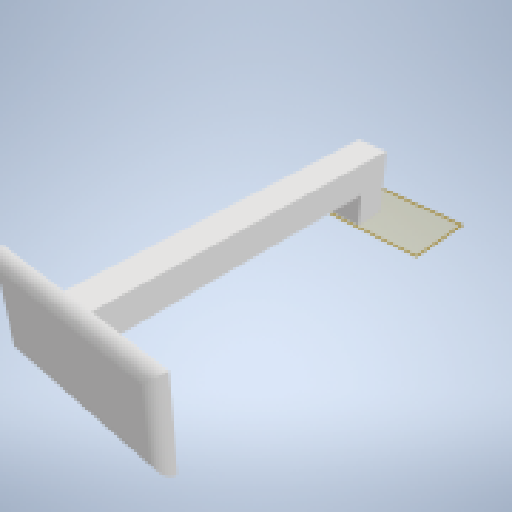
# Autodesk Inventor part: Part61
Saved by Autodesk Inventor 2023 (Build 270158000, 158)
## iProperties
Created: 2023-02-13
Part Number: Part61
Material: Generic
Document SubType Name: Modeling
Designer: klebe
Density: 1 g/cm^3
Appearance: Default
Author: klebe
Autodesk Inventor part; units mm, degrees
ref_plane "YZ Plane" through (0, 0, 0) normal (1, 0, 0) x (0, 1, 0)
ref_plane "XZ Plane" through (0, 0, 0) normal (0, 1, 0) x (-1, 0, 0)
ref_plane "XY Plane" through (0, 0, 0) normal (0, 0, 1) x (1, 0, 0)
ref_plane "Work Plane1" through (-0.3785, 403, -180) normal (0, 1, 0) x (-1, 0, 0)
sketch "Sketch1" plane through (-0.3785, 403, -180) normal (0, 1, 0) x (-1, 0, 0)
  line L0 (545.5132, 110) -> (570.5132, 110)
  line L1 (570.5132, 110) -> (570.5132, 60)
  line L2 (570.5132, 60) -> (545.5132, 60)
  line L3 (545.5132, 60) -> (520.5132, 60)
  line L4 (520.5132, 60) -> (520.5132, 110)
  line L5 (520.5132, 110) -> (545.5132, 110)
  point P0 (-0.3785, 180)
  dimension "d2" = 25
  dimension "d3" = 25
  constraints: 12 end point, 2 horizontal, 2 parallel, 2 perpendicular, 1 point on line
  measures "d2" distance of L1.end L2.end
  measures "d3" distance of L4.end L5.end
extrude "Extrusion1" add sketch "Sketch1" along normal blind 50
sketch "Sketch2" plane through (-520.8916, 403, -120) normal (0, 0, -1) x (-1, 0, 0)
  line L0 (50, 50) -> (0, 50) projected
  line L1 (50, 50) -> (0, 50)
  line L2 (0, 50) -> (0, 100)
  line L3 (0, 100) -> (50, 100)
  line L4 (50, 100) -> (50, 50)
  point P0 (-520.8916, -403)
  dimension "d6" = 50
  constraints: 8 end point, 2 parallel, 1 horizontal, 1 perpendicular
  measures "d6" distance of L1.end L2.end
extrude "Extrusion2" add sketch "Sketch2" against normal blind 500
sketch "Sketch3" plane through (-520.8916, 403, 380) normal (0, 0, 1) x (1, 0, 0)
  line L0 (0, 100) -> (-50, 100) projected
  line L1 (-50, 100) -> (-50, 50) projected
  line L2 (-50, 50) -> (0, 50) projected
  line L3 (0, 50) -> (0, 100) projected
  line L4 (-25, 100) -> (125, 100)
  line L5 (125, 100) -> (-175, 100)
  line L6 (-175, 100) -> (-175, -50)
  line L7 (-175, -50) -> (125, -50)
  line L8 (125, -50) -> (125, 100)
  point P0 (520.8916, -403)
  dimension "d9" = 150
  dimension "d10" = 300
  dimension "d11" = 150
  constraints: 10 end point, 2 horizontal, 2 parallel, 1 midpoint, 1 perpendicular
  measures "d9" distance of L4.start L4.end
  measures "d10" distance of L7.end L6.end
  measures "d11" distance of L6.end L5.end
extrude "Extrusion3" add sketch "Sketch3" along normal blind 20
fillet "Fillet1" radius 20 3 edges at (-695.8916, 428, 400) (-545.8916, 353, 400) (-395.8916, 428, 400)
body "Solid1"
